Autodesk Inventor part; units mm, degrees
note: some values were not read from the file. Chosen so that the rebuilt part matches the saved one: sketch regions of "Extrusion4".
(part 2 of 2)
sketch "Skizze14" plane through (0, 0, -25) normal (0, 0, -1) x (-1, 0, 0)
  circle A0 centre (0, 0) radius 27.4555 construction
  circle A1 centre (0, 0) radius 26.4655
  circle A2 centre (0, 0) radius 29.1655 construction
  circle A3 centre (0, 0) radius 27.2155 construction
  line L0 (-1.465, 27.176) -> (1.465, 27.176) construction
  line L1 (3.028, 27.0465) -> (5.918, 26.5643) construction
  arc A4 (4.0071, 28.7853) -> (3.1451, 27.5107) centre (5.918, 26.5643) ccw
  arc A5 (0.5608, 29.1601) -> (0, 29.1655) centre (0, 0) ccw
  arc A6 (4.8005, 28.7677) -> (4.2464, 28.8547) centre (0, 0) ccw
  arc A7 (2.8303, 27.3092) -> (1.7033, 27.4026) centre (0, 0) ccw
  arc A8 (1.4259, 27.6532) -> (0.7855, 29.0523) centre (-1.465, 27.176) ccw
  arc A9 (0.7855, 29.0523) -> (0.5608, 29.1601) centre (0.5551, 28.8602) ccw
  arc A10 (1.4259, 27.6532) -> (1.7033, 27.4026) centre (1.7219, 27.702) ccw
  arc A11 (2.8303, 27.3092) -> (3.1451, 27.5107) centre (2.8612, 27.6076) ccw
  arc A12 (4.2464, 28.8547) -> (4.0071, 28.7853) centre (4.2027, 28.5579) ccw
  line L2 (-49.6175, 0) -> (49.6175, 0) construction
  line L3 (0, -54.7) -> (0, 48.2) construction
  line L4 (4.8005, 28.7677) -> (0, 0) construction
  line L5 (0, 0) -> (2.5656, 30.9622) construction
  arc A13 (-0.5608, 29.1601) -> (-0.7855, 29.0523) centre (-0.5551, 28.8602) ccw
  arc A14 (-0.7855, 29.0523) -> (-1.4259, 27.6532) centre (1.465, 27.176) ccw
  arc A15 (-1.7033, 27.4026) -> (-1.4259, 27.6532) centre (-1.7219, 27.702) ccw
  arc A16 (-3.1451, 27.5107) -> (-2.8303, 27.3092) centre (-2.8612, 27.6076) ccw
  arc A17 (-3.1451, 27.5107) -> (-4.0071, 28.7853) centre (-5.918, 26.5643) ccw
  arc A18 (-4.0071, 28.7853) -> (-4.2464, 28.8547) centre (-4.2027, 28.5579) ccw
  arc A19 (0, 29.1655) -> (-0.5608, 29.1601) centre (0, 0) ccw
  arc A20 (-4.2464, 28.8547) -> (-4.8005, 28.7677) centre (0, 0) ccw
  arc A21 (-1.7033, 27.4026) -> (-2.8303, 27.3092) centre (0, 0) ccw
  arc A22 (-5.3528, 28.6701) -> (-5.5566, 28.5267) centre (-5.2977, 28.3752) ccw
  arc A23 (-5.5566, 28.5267) -> (-5.958, 27.0413) centre (-3.028, 27.0465) ccw
  arc A24 (-6.1904, 26.7485) -> (-5.958, 27.0413) centre (-6.258, 27.0408) ccw
  arc A25 (-7.6303, 26.6178) -> (-7.2866, 26.4709) centre (-7.3662, 26.7602) ccw
  arc A26 (-7.6303, 26.6178) -> (-8.6903, 27.7332) centre (-10.2097, 25.2279) ccw
  arc A27 (-8.6903, 27.7332) -> (-8.9378, 27.7622) centre (-8.8459, 27.4767) ccw
  arc A28 (-4.8005, 28.7677) -> (-5.3528, 28.6701) centre (0, 0) ccw
  arc A29 (-8.9378, 27.7622) -> (-9.47, 27.5852) centre (0, 0) ccw
  arc A30 (-6.1904, 26.7485) -> (-7.2866, 26.4709) centre (0, 0) ccw
  arc A31 (-9.9987, 27.398) -> (-10.1762, 27.2231) centre (-9.8959, 27.1162) ccw
  arc A32 (-10.1762, 27.2231) -> (-10.3276, 25.6919) centre (-7.4384, 26.1792) ccw
  arc A33 (-10.5086, 25.3648) -> (-10.3276, 25.6919) centre (-10.6234, 25.642) ccw
  arc A34 (-11.9074, 24.9989) -> (-11.5442, 24.9105) centre (-11.6704, 25.1827) ccw
  arc A35 (-11.9074, 24.9989) -> (-13.1365, 25.9246) centre (-14.2228, 23.2033) ccw
  arc A36 (-13.1365, 25.9246) -> (-13.3854, 25.9125) centre (-13.2478, 25.6459) ccw
  arc A37 (-9.47, 27.5852) -> (-9.9987, 27.398) centre (0, 0) ccw
  arc A38 (-13.3854, 25.9125) -> (-13.8812, 25.6503) centre (0, 0) ccw
  arc A39 (-10.5086, 25.3648) -> (-11.5442, 24.9105) centre (0, 0) ccw
  arc A40 (-14.3719, 25.3786) -> (-14.5182, 25.1769) centre (-14.2241, 25.1176) ccw
  arc A41 (-14.5182, 25.1769) -> (-14.4155, 23.6416) centre (-11.6459, 24.5979) ccw
  arc A42 (-14.5402, 23.2892) -> (-14.4155, 23.6416) centre (-14.6991, 23.5437) ccw
  arc A43 (-15.8597, 22.698) -> (-15.4869, 22.6707) centre (-15.6561, 22.9184) ccw
  arc A44 (-15.8597, 22.698) -> (-17.2244, 23.4088) centre (-17.848, 20.5459) ccw
  arc A45 (-17.2244, 23.4088) -> (-17.4679, 23.3559) centre (-17.2883, 23.1156) ccw
  arc A46 (-13.8812, 25.6503) -> (-14.3719, 25.3786) centre (0, 0) ccw
  arc A47 (-17.4679, 23.3559) -> (-17.9138, 23.0157) centre (0, 0) ccw
  arc A48 (-14.5402, 23.2892) -> (-15.4869, 22.6707) centre (0, 0) ccw
  arc A49 (-18.3531, 22.667) -> (-18.4641, 22.4439) centre (-18.1643, 22.4338) ccw
  arc A50 (-18.4641, 22.4439) -> (-18.1102, 20.9464) centre (-15.5358, 22.3455) ccw
  arc A51 (-18.1752, 20.5783) -> (-18.1102, 20.9464) centre (-18.3737, 20.8032) ccw
  arc A52 (-19.3794, 19.778) -> (-19.0072, 19.8124) centre (-19.2148, 20.0289) ccw
  arc A53 (-19.3794, 19.778) -> (-20.8425, 20.2545) centre (-20.9863, 17.328) ccw
  arc A54 (-20.8425, 20.2545) -> (-21.0739, 20.1622) centre (-20.8572, 19.9548) ccw
  arc A55 (-17.9138, 23.0157) -> (-18.3531, 22.667) centre (0, 0) ccw
  arc A56 (-21.0739, 20.1622) -> (-21.4578, 19.7533) centre (0, 0) ccw
  arc A57 (-18.1752, 20.5783) -> (-19.0072, 19.8124) centre (0, 0) ccw
  arc A58 (-21.8336, 19.337) -> (-21.9064, 19.0987) centre (-21.609, 19.1381) ccw
  arc A59 (-21.9064, 19.0987) -> (-21.3108, 17.6799) centre (-19.0018, 19.4837) ccw
  arc A60 (-21.3144, 17.3061) -> (-21.3108, 17.6799) centre (-21.5472, 17.4952) ccw
  arc A61 (-22.3704, 16.3186) -> (-22.0089, 16.4137) centre (-22.2494, 16.5931) ccw
  arc A62 (-22.3704, 16.3186) -> (-23.892, 16.5477) centre (-23.5521, 13.6374) ccw
  arc A63 (-23.892, 16.5477) -> (-24.1051, 16.4186) centre (-23.8572, 16.2497) ccw
  arc A64 (-21.4578, 19.7533) -> (-21.8336, 19.337) centre (0, 0) ccw
  arc A65 (-24.1051, 16.4186) -> (-24.4164, 15.952) centre (0, 0) ccw
  arc A66 (-21.3144, 17.3061) -> (-22.0089, 16.4137) centre (0, 0) ccw
  arc A67 (-24.7186, 15.4796) -> (-24.7512, 15.2325) centre (-24.4643, 15.3203) ccw
  arc A68 (-24.7512, 15.2325) -> (-23.9302, 13.9311) centre (-21.9496, 16.0903) ccw
  arc A69 (-23.8721, 13.5619) -> (-23.9302, 13.9311) centre (-24.133, 13.7101) ccw
  arc A70 (-24.7513, 12.4139) -> (-24.4104, 12.5673) centre (-24.6771, 12.7046) ccw
  arc A71 (-24.7513, 12.4139) -> (-26.2898, 12.3895) centre (-25.4756, 9.5749) ccw
  arc A72 (-26.2898, 12.3895) -> (-26.4788, 12.2271) centre (-26.2064, 12.1013) ccw
  arc A73 (-24.4164, 15.952) -> (-24.7186, 15.4796) centre (0, 0) ccw
  arc A74 (-26.4788, 12.2271) -> (-26.709, 11.7156) centre (0, 0) ccw
  arc A75 (-23.8721, 13.5619) -> (-24.4104, 12.5673) centre (0, 0) ccw
  arc A76 (-26.9293, 11.1999) -> (-26.9208, 10.9508) centre (-26.6523, 11.0847) ccw
  arc A77 (-26.9208, 10.9508) -> (-25.8968, 9.8024) centre (-24.2986, 12.2581) ccw
  arc A78 (-25.7788, 9.4477) -> (-25.8968, 9.8024) centre (-26.0605, 9.5509) ccw
  arc A79 (-26.457, 8.1707) -> (-26.146, 8.3781) centre (-26.4317, 8.4696) ccw
  arc A80 (-26.457, 8.1707) -> (-27.9704, 7.8934) centre (-26.7041, 5.2512) ccw
  arc A81 (-27.9704, 7.8934) -> (-28.1301, 7.702) centre (-27.8408, 7.6228) ccw
  arc A82 (-26.709, 11.7156) -> (-26.9293, 11.1999) centre (0, 0) ccw
  arc A83 (-28.1301, 7.702) -> (-28.273, 7.1597) centre (0, 0) ccw
  arc A84 (-25.7788, 9.4477) -> (-26.146, 8.3781) centre (0, 0) ccw
  arc A85 (-28.4055, 6.6147) -> (-28.3561, 6.3705) centre (-28.1133, 6.5467) ccw
  arc A86 (-28.3561, 6.3705) -> (-27.157, 5.4062) centre (-25.9848, 8.0915) ccw
  arc A87 (-26.9822, 5.0758) -> (-27.157, 5.4062) centre (-27.2771, 5.1313) ccw
  arc A88 (-27.441, 3.7046) -> (-27.1684, 3.9603) centre (-27.4652, 4.0036) ccw
  arc A89 (-27.441, 3.7046) -> (-28.8882, 3.1819) centre (-27.2042, 0.7842) ccw
  arc A90 (-28.8882, 3.1819) -> (-29.0142, 2.9669) centre (-28.7157, 2.9364) ccw
  arc A91 (-28.273, 7.1597) -> (-28.4055, 6.6147) centre (0, 0) ccw
  arc A92 (-29.0142, 2.9669) -> (-29.0659, 2.4085) centre (0, 0) ccw
  arc A93 (-26.9822, 5.0758) -> (-27.1684, 3.9603) centre (0, 0) ccw
  arc A94 (-29.1068, 1.8491) -> (-29.0179, 1.6163) centre (-28.8074, 1.8301) ccw
  arc A95 (-29.0179, 1.6163) -> (-27.6765, 0.8626) centre (-26.9622, 3.7042) ccw
  arc A96 (-27.4497, 0.5654) -> (-27.6765, 0.8626) centre (-27.7496, 0.5716) ccw
  arc A97 (-27.6765, -0.8626) -> (-27.4497, -0.5654) centre (-27.7496, -0.5716) ccw
  arc A98 (-27.6765, -0.8626) -> (-29.0179, -1.6163) centre (-26.9622, -3.7042) ccw
  arc A99 (-29.0179, -1.6163) -> (-29.1068, -1.8491) centre (-28.8074, -1.8301) ccw
  arc A100 (-29.0659, 2.4085) -> (-29.1068, 1.8491) centre (0, 0) ccw
  arc A101 (-29.1068, -1.8491) -> (-29.0659, -2.4085) centre (0, 0) ccw
  arc A102 (-27.4497, 0.5654) -> (-27.4497, -0.5654) centre (0, 0) ccw
  arc A103 (-29.0142, -2.9669) -> (-28.8882, -3.1819) centre (-28.7157, -2.9364) ccw
  arc A104 (-28.8882, -3.1819) -> (-27.441, -3.7046) centre (-27.2042, -0.7842) ccw
  arc A105 (-27.1684, -3.9603) -> (-27.441, -3.7046) centre (-27.4652, -4.0036) ccw
  arc A106 (-27.157, -5.4062) -> (-26.9822, -5.0758) centre (-27.2771, -5.1313) ccw
  arc A107 (-27.157, -5.4062) -> (-28.3561, -6.3705) centre (-25.9848, -8.0915) ccw
  arc A108 (-28.3561, -6.3705) -> (-28.4055, -6.6147) centre (-28.1133, -6.5467) ccw
  arc A109 (-29.0659, -2.4085) -> (-29.0142, -2.9669) centre (0, 0) ccw
  arc A110 (-28.4055, -6.6147) -> (-28.273, -7.1597) centre (0, 0) ccw
  arc A111 (-27.1684, -3.9603) -> (-26.9822, -5.0758) centre (0, 0) ccw
  arc A112 (-28.1301, -7.702) -> (-27.9704, -7.8934) centre (-27.8408, -7.6228) ccw
  arc A113 (-27.9704, -7.8934) -> (-26.457, -8.1707) centre (-26.7041, -5.2512) ccw
  arc A114 (-26.146, -8.3781) -> (-26.457, -8.1707) centre (-26.4317, -8.4696) ccw
  arc A115 (-25.8968, -9.8024) -> (-25.7788, -9.4477) centre (-26.0605, -9.5509) ccw
  arc A116 (-25.8968, -9.8024) -> (-26.9208, -10.9508) centre (-24.2986, -12.2581) ccw
  arc A117 (-26.9208, -10.9508) -> (-26.9293, -11.1999) centre (-26.6523, -11.0847) ccw
  arc A118 (-28.273, -7.1597) -> (-28.1301, -7.702) centre (0, 0) ccw
  arc A119 (-26.9293, -11.1999) -> (-26.709, -11.7156) centre (0, 0) ccw
  arc A120 (-26.146, -8.3781) -> (-25.7788, -9.4477) centre (0, 0) ccw
  arc A121 (-26.4788, -12.2271) -> (-26.2898, -12.3895) centre (-26.2064, -12.1013) ccw
  arc A122 (-26.2898, -12.3895) -> (-24.7513, -12.4139) centre (-25.4756, -9.5749) ccw
  arc A123 (-24.4104, -12.5673) -> (-24.7513, -12.4139) centre (-24.6771, -12.7046) ccw
  arc A124 (-23.9302, -13.9311) -> (-23.8721, -13.5619) centre (-24.133, -13.7101) ccw
  arc A125 (-23.9302, -13.9311) -> (-24.7512, -15.2325) centre (-21.9496, -16.0903) ccw
  arc A126 (-24.7512, -15.2325) -> (-24.7186, -15.4796) centre (-24.4643, -15.3203) ccw
  arc A127 (-26.709, -11.7156) -> (-26.4788, -12.2271) centre (0, 0) ccw
  arc A128 (-24.7186, -15.4796) -> (-24.4164, -15.952) centre (0, 0) ccw
  arc A129 (-24.4104, -12.5673) -> (-23.8721, -13.5619) centre (0, 0) ccw
  arc A130 (-24.1051, -16.4186) -> (-23.892, -16.5477) centre (-23.8572, -16.2497) ccw
  arc A131 (-23.892, -16.5477) -> (-22.3704, -16.3186) centre (-23.5521, -13.6374) ccw
  arc A132 (-22.0089, -16.4137) -> (-22.3704, -16.3186) centre (-22.2494, -16.5931) ccw
  arc A133 (-21.3108, -17.6799) -> (-21.3144, -17.3061) centre (-21.5472, -17.4952) ccw
  arc A134 (-21.3108, -17.6799) -> (-21.9064, -19.0987) centre (-19.0018, -19.4837) ccw
  arc A135 (-21.9064, -19.0987) -> (-21.8336, -19.337) centre (-21.609, -19.1381) ccw
  arc A136 (-24.4164, -15.952) -> (-24.1051, -16.4186) centre (0, 0) ccw
  arc A137 (-21.8336, -19.337) -> (-21.4578, -19.7533) centre (0, 0) ccw
  arc A138 (-22.0089, -16.4137) -> (-21.3144, -17.3061) centre (0, 0) ccw
  arc A139 (-21.0739, -20.1622) -> (-20.8425, -20.2545) centre (-20.8572, -19.9548) ccw
  arc A140 (-20.8425, -20.2545) -> (-19.3794, -19.778) centre (-20.9863, -17.328) ccw
  arc A141 (-19.0072, -19.8124) -> (-19.3794, -19.778) centre (-19.2148, -20.0289) ccw
  arc A142 (-18.1102, -20.9464) -> (-18.1752, -20.5783) centre (-18.3737, -20.8032) ccw
  arc A143 (-18.1102, -20.9464) -> (-18.4641, -22.4439) centre (-15.5358, -22.3455) ccw
  arc A144 (-18.4641, -22.4439) -> (-18.3531, -22.667) centre (-18.1643, -22.4338) ccw
  arc A145 (-21.4578, -19.7533) -> (-21.0739, -20.1622) centre (0, 0) ccw
  arc A146 (-18.3531, -22.667) -> (-17.9138, -23.0157) centre (0, 0) ccw
  arc A147 (-19.0072, -19.8124) -> (-18.1752, -20.5783) centre (0, 0) ccw
  arc A148 (-17.4679, -23.3559) -> (-17.2244, -23.4088) centre (-17.2883, -23.1156) ccw
  arc A149 (-17.2244, -23.4088) -> (-15.8597, -22.698) centre (-17.848, -20.5459) ccw
  arc A150 (-15.4869, -22.6707) -> (-15.8597, -22.698) centre (-15.6561, -22.9184) ccw
  arc A151 (-14.4155, -23.6416) -> (-14.5402, -23.2892) centre (-14.6991, -23.5437) ccw
  arc A152 (-14.4155, -23.6416) -> (-14.5182, -25.1769) centre (-11.6459, -24.5979) ccw
  arc A153 (-14.5182, -25.1769) -> (-14.3719, -25.3786) centre (-14.2241, -25.1176) ccw
  arc A154 (-17.9138, -23.0157) -> (-17.4679, -23.3559) centre (0, 0) ccw
  arc A155 (-14.3719, -25.3786) -> (-13.8812, -25.6503) centre (0, 0) ccw
  arc A156 (-15.4869, -22.6707) -> (-14.5402, -23.2892) centre (0, 0) ccw
  arc A157 (-13.3854, -25.9125) -> (-13.1365, -25.9246) centre (-13.2478, -25.6459) ccw
  arc A158 (-13.1365, -25.9246) -> (-11.9074, -24.9989) centre (-14.2228, -23.2033) ccw
  arc A159 (-11.5442, -24.9105) -> (-11.9074, -24.9989) centre (-11.6704, -25.1827) ccw
  arc A160 (-10.3276, -25.6919) -> (-10.5086, -25.3648) centre (-10.6234, -25.642) ccw
  arc A161 (-10.3276, -25.6919) -> (-10.1762, -27.2231) centre (-7.4384, -26.1792) ccw
  arc A162 (-10.1762, -27.2231) -> (-9.9987, -27.398) centre (-9.8959, -27.1162) ccw
  arc A163 (-13.8812, -25.6503) -> (-13.3854, -25.9125) centre (0, 0) ccw
  arc A164 (-9.9987, -27.398) -> (-9.47, -27.5852) centre (0, 0) ccw
  arc A165 (-11.5442, -24.9105) -> (-10.5086, -25.3648) centre (0, 0) ccw
  arc A166 (-8.9378, -27.7622) -> (-8.6903, -27.7332) centre (-8.8459, -27.4767) ccw
  arc A167 (-8.6903, -27.7332) -> (-7.6303, -26.6178) centre (-10.2097, -25.2279) ccw
  arc A168 (-7.2866, -26.4709) -> (-7.6303, -26.6178) centre (-7.3662, -26.7602) ccw
  arc A169 (-5.958, -27.0413) -> (-6.1904, -26.7485) centre (-6.258, -27.0408) ccw
  arc A170 (-5.958, -27.0413) -> (-5.5566, -28.5267) centre (-3.028, -27.0465) ccw
  arc A171 (-5.5566, -28.5267) -> (-5.3528, -28.6701) centre (-5.2977, -28.3752) ccw
  arc A172 (-9.47, -27.5852) -> (-8.9378, -27.7622) centre (0, 0) ccw
  arc A173 (-5.3528, -28.6701) -> (-4.8005, -28.7677) centre (0, 0) ccw
  arc A174 (-7.2866, -26.4709) -> (-6.1904, -26.7485) centre (0, 0) ccw
  arc A175 (-4.2464, -28.8547) -> (-4.0071, -28.7853) centre (-4.2027, -28.5579) ccw
  arc A176 (-4.0071, -28.7853) -> (-3.1451, -27.5107) centre (-5.918, -26.5643) ccw
  arc A177 (-2.8303, -27.3092) -> (-3.1451, -27.5107) centre (-2.8612, -27.6076) ccw
  arc A178 (-1.4259, -27.6532) -> (-1.7033, -27.4026) centre (-1.7219, -27.702) ccw
  arc A179 (-1.4259, -27.6532) -> (-0.7855, -29.0523) centre (1.465, -27.176) ccw
  arc A180 (-0.7855, -29.0523) -> (-0.5608, -29.1601) centre (-0.5551, -28.8602) ccw
  arc A181 (-4.8005, -28.7677) -> (-4.2464, -28.8547) centre (0, 0) ccw
  arc A182 (-0.5608, -29.1601) -> (0, -29.1655) centre (0, 0) ccw
  arc A183 (-2.8303, -27.3092) -> (-1.7033, -27.4026) centre (0, 0) ccw
  arc A184 (0.5608, -29.1601) -> (0.7855, -29.0523) centre (0.5551, -28.8602) ccw
  arc A185 (0.7855, -29.0523) -> (1.4259, -27.6532) centre (-1.465, -27.176) ccw
  arc A186 (1.7033, -27.4026) -> (1.4259, -27.6532) centre (1.7219, -27.702) ccw
  arc A187 (3.1451, -27.5107) -> (2.8303, -27.3092) centre (2.8612, -27.6076) ccw
  arc A188 (3.1451, -27.5107) -> (4.0071, -28.7853) centre (5.918, -26.5643) ccw
  arc A189 (4.0071, -28.7853) -> (4.2464, -28.8547) centre (4.2027, -28.5579) ccw
  arc A190 (0, -29.1655) -> (0.5608, -29.1601) centre (0, 0) ccw
  arc A191 (4.2464, -28.8547) -> (4.8005, -28.7677) centre (0, 0) ccw
  arc A192 (1.7033, -27.4026) -> (2.8303, -27.3092) centre (0, 0) ccw
  arc A193 (5.3528, -28.6701) -> (5.5566, -28.5267) centre (5.2977, -28.3752) ccw
  arc A194 (5.5566, -28.5267) -> (5.958, -27.0413) centre (3.028, -27.0465) ccw
  arc A195 (6.1904, -26.7485) -> (5.958, -27.0413) centre (6.258, -27.0408) ccw
  arc A196 (7.6303, -26.6178) -> (7.2866, -26.4709) centre (7.3662, -26.7602) ccw
  arc A197 (7.6303, -26.6178) -> (8.6903, -27.7332) centre (10.2097, -25.2279) ccw
  arc A198 (8.6903, -27.7332) -> (8.9378, -27.7622) centre (8.8459, -27.4767) ccw
  arc A199 (4.8005, -28.7677) -> (5.3528, -28.6701) centre (0, 0) ccw
  arc A200 (8.9378, -27.7622) -> (9.47, -27.5852) centre (0, 0) ccw
  arc A201 (6.1904, -26.7485) -> (7.2866, -26.4709) centre (0, 0) ccw
  arc A202 (9.9987, -27.398) -> (10.1762, -27.2231) centre (9.8959, -27.1162) ccw
  arc A203 (10.1762, -27.2231) -> (10.3276, -25.6919) centre (7.4384, -26.1792) ccw
  arc A204 (10.5086, -25.3648) -> (10.3276, -25.6919) centre (10.6234, -25.642) ccw
  arc A205 (11.9074, -24.9989) -> (11.5442, -24.9105) centre (11.6704, -25.1827) ccw
  arc A206 (11.9074, -24.9989) -> (13.1365, -25.9246) centre (14.2228, -23.2033) ccw
  arc A207 (13.1365, -25.9246) -> (13.3854, -25.9125) centre (13.2478, -25.6459) ccw
  arc A208 (9.47, -27.5852) -> (9.9987, -27.398) centre (0, 0) ccw
  arc A209 (13.3854, -25.9125) -> (13.8812, -25.6503) centre (0, 0) ccw
  arc A210 (10.5086, -25.3648) -> (11.5442, -24.9105) centre (0, 0) ccw
  arc A211 (14.3719, -25.3786) -> (14.5182, -25.1769) centre (14.2241, -25.1176) ccw
  arc A212 (14.5182, -25.1769) -> (14.4155, -23.6416) centre (11.6459, -24.5979) ccw
  arc A213 (14.5402, -23.2892) -> (14.4155, -23.6416) centre (14.6991, -23.5437) ccw
  arc A214 (15.8597, -22.698) -> (15.4869, -22.6707) centre (15.6561, -22.9184) ccw
  arc A215 (15.8597, -22.698) -> (17.2244, -23.4088) centre (17.848, -20.5459) ccw
  arc A216 (17.2244, -23.4088) -> (17.4679, -23.3559) centre (17.2883, -23.1156) ccw
  arc A217 (13.8812, -25.6503) -> (14.3719, -25.3786) centre (0, 0) ccw
  arc A218 (17.4679, -23.3559) -> (17.9138, -23.0157) centre (0, 0) ccw
  arc A219 (14.5402, -23.2892) -> (15.4869, -22.6707) centre (0, 0) ccw
  arc A220 (18.3531, -22.667) -> (18.4641, -22.4439) centre (18.1643, -22.4338) ccw
  arc A221 (18.4641, -22.4439) -> (18.1102, -20.9464) centre (15.5358, -22.3455) ccw
  arc A222 (18.1752, -20.5783) -> (18.1102, -20.9464) centre (18.3737, -20.8032) ccw
  arc A223 (19.3794, -19.778) -> (19.0072, -19.8124) centre (19.2148, -20.0289) ccw
  arc A224 (19.3794, -19.778) -> (20.8425, -20.2545) centre (20.9863, -17.328) ccw
  arc A225 (20.8425, -20.2545) -> (21.0739, -20.1622) centre (20.8572, -19.9548) ccw
  arc A226 (17.9138, -23.0157) -> (18.3531, -22.667) centre (0, 0) ccw
  arc A227 (21.0739, -20.1622) -> (21.4578, -19.7533) centre (0, 0) ccw
  arc A228 (18.1752, -20.5783) -> (19.0072, -19.8124) centre (0, 0) ccw
  arc A229 (21.8336, -19.337) -> (21.9064, -19.0987) centre (21.609, -19.1381) ccw
  arc A230 (21.9064, -19.0987) -> (21.3108, -17.6799) centre (19.0018, -19.4837) ccw
  arc A231 (21.3144, -17.3061) -> (21.3108, -17.6799) centre (21.5472, -17.4952) ccw
  arc A232 (22.3704, -16.3186) -> (22.0089, -16.4137) centre (22.2494, -16.5931) ccw
  arc A233 (22.3704, -16.3186) -> (23.892, -16.5477) centre (23.5521, -13.6374) ccw
  arc A234 (23.892, -16.5477) -> (24.1051, -16.4186) centre (23.8572, -16.2497) ccw
  arc A235 (21.4578, -19.7533) -> (21.8336, -19.337) centre (0, 0) ccw
  arc A236 (24.1051, -16.4186) -> (24.4164, -15.952) centre (0, 0) ccw
  arc A237 (21.3144, -17.3061) -> (22.0089, -16.4137) centre (0, 0) ccw
  arc A238 (24.7186, -15.4796) -> (24.7512, -15.2325) centre (24.4643, -15.3203) ccw
  arc A239 (24.7512, -15.2325) -> (23.9302, -13.9311) centre (21.9496, -16.0903) ccw
  arc A240 (23.8721, -13.5619) -> (23.9302, -13.9311) centre (24.133, -13.7101) ccw
  arc A241 (24.7513, -12.4139) -> (24.4104, -12.5673) centre (24.6771, -12.7046) ccw
  arc A242 (24.7513, -12.4139) -> (26.2898, -12.3895) centre (25.4756, -9.5749) ccw
  arc A243 (26.2898, -12.3895) -> (26.4788, -12.2271) centre (26.2064, -12.1013) ccw
  arc A244 (24.4164, -15.952) -> (24.7186, -15.4796) centre (0, 0) ccw
  arc A245 (26.4788, -12.2271) -> (26.709, -11.7156) centre (0, 0) ccw
  arc A246 (23.8721, -13.5619) -> (24.4104, -12.5673) centre (0, 0) ccw
  arc A247 (26.9293, -11.1999) -> (26.9208, -10.9508) centre (26.6523, -11.0847) ccw
  arc A248 (26.9208, -10.9508) -> (25.8968, -9.8024) centre (24.2986, -12.2581) ccw
  arc A249 (25.7788, -9.4477) -> (25.8968, -9.8024) centre (26.0605, -9.5509) ccw
  arc A250 (26.457, -8.1707) -> (26.146, -8.3781) centre (26.4317, -8.4696) ccw
  arc A251 (26.457, -8.1707) -> (27.9704, -7.8934) centre (26.7041, -5.2512) ccw
  arc A252 (27.9704, -7.8934) -> (28.1301, -7.702) centre (27.8408, -7.6228) ccw
  arc A253 (26.709, -11.7156) -> (26.9293, -11.1999) centre (0, 0) ccw
  arc A254 (28.1301, -7.702) -> (28.273, -7.1597) centre (0, 0) ccw
  arc A255 (25.7788, -9.4477) -> (26.146, -8.3781) centre (0, 0) ccw
  arc A256 (28.4055, -6.6147) -> (28.3561, -6.3705) centre (28.1133, -6.5467) ccw
  arc A257 (28.3561, -6.3705) -> (27.157, -5.4062) centre (25.9848, -8.0915) ccw
  arc A258 (26.9822, -5.0758) -> (27.157, -5.4062) centre (27.2771, -5.1313) ccw
  arc A259 (27.441, -3.7046) -> (27.1684, -3.9603) centre (27.4652, -4.0036) ccw
  arc A260 (27.441, -3.7046) -> (28.8882, -3.1819) centre (27.2042, -0.7842) ccw
  arc A261 (28.8882, -3.1819) -> (29.0142, -2.9669) centre (28.7157, -2.9364) ccw
  arc A262 (28.273, -7.1597) -> (28.4055, -6.6147) centre (0, 0) ccw
  arc A263 (29.0142, -2.9669) -> (29.0659, -2.4085) centre (0, 0) ccw
  arc A264 (26.9822, -5.0758) -> (27.1684, -3.9603) centre (0, 0) ccw
  arc A265 (29.1068, -1.8491) -> (29.0179, -1.6163) centre (28.8074, -1.8301) ccw
  arc A266 (29.0179, -1.6163) -> (27.6765, -0.8626) centre (26.9622, -3.7042) ccw
  arc A267 (27.4497, -0.5654) -> (27.6765, -0.8626) centre (27.7496, -0.5716) ccw
  arc A268 (27.6765, 0.8626) -> (27.4497, 0.5654) centre (27.7496, 0.5716) ccw
  arc A269 (27.6765, 0.8626) -> (29.0179, 1.6163) centre (26.9622, 3.7042) ccw
  arc A270 (29.0179, 1.6163) -> (29.1068, 1.8491) centre (28.8074, 1.8301) ccw
  arc A271 (29.0659, -2.4085) -> (29.1068, -1.8491) centre (0, 0) ccw
  arc A272 (29.1068, 1.8491) -> (29.0659, 2.4085) centre (0, 0) ccw
  arc A273 (27.4497, -0.5654) -> (27.4497, 0.5654) centre (0, 0) ccw
  arc A274 (29.0142, 2.9669) -> (28.8882, 3.1819) centre (28.7157, 2.9364) ccw
  arc A275 (28.8882, 3.1819) -> (27.441, 3.7046) centre (27.2042, 0.7842) ccw
  arc A276 (27.1684, 3.9603) -> (27.441, 3.7046) centre (27.4652, 4.0036) ccw
  arc A277 (27.157, 5.4062) -> (26.9822, 5.0758) centre (27.2771, 5.1313) ccw
  arc A278 (27.157, 5.4062) -> (28.3561, 6.3705) centre (25.9848, 8.0915) ccw
  arc A279 (28.3561, 6.3705) -> (28.4055, 6.6147) centre (28.1133, 6.5467) ccw
  arc A280 (29.0659, 2.4085) -> (29.0142, 2.9669) centre (0, 0) ccw
  arc A281 (28.4055, 6.6147) -> (28.273, 7.1597) centre (0, 0) ccw
  arc A282 (27.1684, 3.9603) -> (26.9822, 5.0758) centre (0, 0) ccw
  arc A283 (28.1301, 7.702) -> (27.9704, 7.8934) centre (27.8408, 7.6228) ccw
  arc A284 (27.9704, 7.8934) -> (26.457, 8.1707) centre (26.7041, 5.2512) ccw
  arc A285 (26.146, 8.3781) -> (26.457, 8.1707) centre (26.4317, 8.4696) ccw
  arc A286 (25.8968, 9.8024) -> (25.7788, 9.4477) centre (26.0605, 9.5509) ccw
  arc A287 (25.8968, 9.8024) -> (26.9208, 10.9508) centre (24.2986, 12.2581) ccw
  arc A288 (26.9208, 10.9508) -> (26.9293, 11.1999) centre (26.6523, 11.0847) ccw
  arc A289 (28.273, 7.1597) -> (28.1301, 7.702) centre (0, 0) ccw
  arc A290 (26.9293, 11.1999) -> (26.709, 11.7156) centre (0, 0) ccw
  arc A291 (26.146, 8.3781) -> (25.7788, 9.4477) centre (0, 0) ccw
  arc A292 (26.4788, 12.2271) -> (26.2898, 12.3895) centre (26.2064, 12.1013) ccw
  arc A293 (26.2898, 12.3895) -> (24.7513, 12.4139) centre (25.4756, 9.5749) ccw
  arc A294 (24.4104, 12.5673) -> (24.7513, 12.4139) centre (24.6771, 12.7046) ccw
  arc A295 (23.9302, 13.9311) -> (23.8721, 13.5619) centre (24.133, 13.7101) ccw
  arc A296 (23.9302, 13.9311) -> (24.7512, 15.2325) centre (21.9496, 16.0903) ccw
  arc A297 (24.7512, 15.2325) -> (24.7186, 15.4796) centre (24.4643, 15.3203) ccw
  arc A298 (26.709, 11.7156) -> (26.4788, 12.2271) centre (0, 0) ccw
  arc A299 (24.7186, 15.4796) -> (24.4164, 15.952) centre (0, 0) ccw
  arc A300 (24.4104, 12.5673) -> (23.8721, 13.5619) centre (0, 0) ccw
  arc A301 (24.1051, 16.4186) -> (23.892, 16.5477) centre (23.8572, 16.2497) ccw
  arc A302 (23.892, 16.5477) -> (22.3704, 16.3186) centre (23.5521, 13.6374) ccw
  arc A303 (22.0089, 16.4137) -> (22.3704, 16.3186) centre (22.2494, 16.5931) ccw
  arc A304 (21.3108, 17.6799) -> (21.3144, 17.3061) centre (21.5472, 17.4952) ccw
  arc A305 (21.3108, 17.6799) -> (21.9064, 19.0987) centre (19.0018, 19.4837) ccw
  arc A306 (21.9064, 19.0987) -> (21.8336, 19.337) centre (21.609, 19.1381) ccw
  arc A307 (24.4164, 15.952) -> (24.1051, 16.4186) centre (0, 0) ccw
  arc A308 (21.8336, 19.337) -> (21.4578, 19.7533) centre (0, 0) ccw
  arc A309 (22.0089, 16.4137) -> (21.3144, 17.3061) centre (0, 0) ccw
  arc A310 (21.0739, 20.1622) -> (20.8425, 20.2545) centre (20.8572, 19.9548) ccw
  arc A311 (20.8425, 20.2545) -> (19.3794, 19.778) centre (20.9863, 17.328) ccw
  arc A312 (19.0072, 19.8124) -> (19.3794, 19.778) centre (19.2148, 20.0289) ccw
  arc A313 (18.1102, 20.9464) -> (18.1752, 20.5783) centre (18.3737, 20.8032) ccw
  arc A314 (18.1102, 20.9464) -> (18.4641, 22.4439) centre (15.5358, 22.3455) ccw
  arc A315 (18.4641, 22.4439) -> (18.3531, 22.667) centre (18.1643, 22.4338) ccw
  arc A316 (21.4578, 19.7533) -> (21.0739, 20.1622) centre (0, 0) ccw
  arc A317 (18.3531, 22.667) -> (17.9138, 23.0157) centre (0, 0) ccw
  arc A318 (19.0072, 19.8124) -> (18.1752, 20.5783) centre (0, 0) ccw
  arc A319 (17.4679, 23.3559) -> (17.2244, 23.4088) centre (17.2883, 23.1156) ccw
  arc A320 (17.2244, 23.4088) -> (15.8597, 22.698) centre (17.848, 20.5459) ccw
  arc A321 (15.4869, 22.6707) -> (15.8597, 22.698) centre (15.6561, 22.9184) ccw
  arc A322 (14.4155, 23.6416) -> (14.5402, 23.2892) centre (14.6991, 23.5437) ccw
  arc A323 (14.4155, 23.6416) -> (14.5182, 25.1769) centre (11.6459, 24.5979) ccw
  arc A324 (14.5182, 25.1769) -> (14.3719, 25.3786) centre (14.2241, 25.1176) ccw
  arc A325 (17.9138, 23.0157) -> (17.4679, 23.3559) centre (0, 0) ccw
  arc A326 (14.3719, 25.3786) -> (13.8812, 25.6503) centre (0, 0) ccw
  arc A327 (15.4869, 22.6707) -> (14.5402, 23.2892) centre (0, 0) ccw
  arc A328 (13.3854, 25.9125) -> (13.1365, 25.9246) centre (13.2478, 25.6459) ccw
  arc A329 (13.1365, 25.9246) -> (11.9074, 24.9989) centre (14.2228, 23.2033) ccw
  arc A330 (11.5442, 24.9105) -> (11.9074, 24.9989) centre (11.6704, 25.1827) ccw
  arc A331 (10.3276, 25.6919) -> (10.5086, 25.3648) centre (10.6234, 25.642) ccw
  arc A332 (10.3276, 25.6919) -> (10.1762, 27.2231) centre (7.4384, 26.1792) ccw
  arc A333 (10.1762, 27.2231) -> (9.9987, 27.398) centre (9.8959, 27.1162) ccw
  arc A334 (13.8812, 25.6503) -> (13.3854, 25.9125) centre (0, 0) ccw
  arc A335 (9.9987, 27.398) -> (9.47, 27.5852) centre (0, 0) ccw
  arc A336 (11.5442, 24.9105) -> (10.5086, 25.3648) centre (0, 0) ccw
  arc A337 (8.9378, 27.7622) -> (8.6903, 27.7332) centre (8.8459, 27.4767) ccw
  arc A338 (8.6903, 27.7332) -> (7.6303, 26.6178) centre (10.2097, 25.2279) ccw
  arc A339 (7.2866, 26.4709) -> (7.6303, 26.6178) centre (7.3662, 26.7602) ccw
  arc A340 (5.958, 27.0413) -> (6.1904, 26.7485) centre (6.258, 27.0408) ccw
  arc A341 (5.958, 27.0413) -> (5.5566, 28.5267) centre (3.028, 27.0465) ccw
  arc A342 (5.5566, 28.5267) -> (5.3528, 28.6701) centre (5.2977, 28.3752) ccw
  arc A343 (9.47, 27.5852) -> (8.9378, 27.7622) centre (0, 0) ccw
  arc A344 (5.3528, 28.6701) -> (4.8005, 28.7677) centre (0, 0) ccw
  arc A345 (7.2866, 26.4709) -> (6.1904, 26.7485) centre (0, 0) ccw
  circle A346 centre (0, 0) radius 30.6655
  circle A347 centre (0, 0) radius 2
  circle A348 centre (0, 0) radius 6.35 construction
  circle A349 centre (0, 6.35) radius 1.5
  circle A350 centre (-6.35, 0) radius 1.5
  circle A351 centre (0, -6.35) radius 1.5
  circle A352 centre (6.35, 0) radius 1.5
  dimension "d298" = 12.7
  dimension "d273" = 1.71
  dimension "d274" = 2.7
  dimension "d275" = 0.75
  dimension "d276" = 54.431
  dimension "d277" = 2.93
  dimension "d278" = 0.3
  dimension "d279" = 2.93
  dimension "d280" = 9.474
  dimension "d291" = 1.5
  dimension "d292" = 4
  dimension "d293" = 3
  dimension "d296" = 360
  constraints: 694 point on circle, 352 centre point, 8 coincident, 8 end point, 8 tangent, 6 equal radius, 2 point on line, 1 equal length, 1 horizontal, 1 vertical alignment, 13 other
  measures "d273" radial gap between concentric circles of A2 A0
  measures "d274" radial gap between concentric circles of A2 A1
  measures "d275" radial gap between concentric circles of A3 A1
  measures "d276" diameter of A3
  measures "d277" distance of L0.start L0.end
  measures "d278" radius of A9
  measures "d279" radius of A8
  measures "d280" angle of L3 L4
  measures "d291" radial gap between concentric circles of A346 A2
  measures "d292" diameter of A347
  measures "d293" diameter of A349
extrude "Extrusion34" add sketch "Skizze14" against normal blind 2 separate body contours A1 | A12 A6 A344 A342 A341 A340 A345 A339 A338 A337 A343 A335 A333 A332 A331 A336 A330 A329 A328 A334 A326 A324 A323 A322 A327 A321 A320 A319 A325 A317 A315 A314 A313 A318 A312 A311 A310 A316 A308 A306 A305 A304 A309 A303 A302 A301 A307 A299 A297 A296 A295 A300 A294 A293 A292 A298 A290 A288 A287 A286 A291 A285 A284 A283 A289 A281 A279 A278 A277 A282 A276 A275 A274 A280 A272 A270 A269 A268 A273 A267 A266 A265 A271 A263 A261 A260 A259 A264 A258 A257 A256 A262 A254 A252 A251 A250 A255 A249 A248 A247 A253 A245 A243 A242 A241 A246 A240 A239 A238 A244 A236 A234 A233 A232 A237 A231 A230 A229 A235 A227 A225 A224 A223 A228 A222 A221 A220 A226 A218 A216 A215 A214 A219 A213 A212 A211 A217 A209 A207 A206 A205 A210 A204 A203 A202 A208 A200 A198 A197 A196 A201 A195 A194 A193 A199 A191 A189 A188 A187 A192 A186 A185 A184 A190 A182 A180 A179 A178 A183 A177 A176 A175 A181 A173 A171 A170 A169 A174 A168 A167 A166 A172 A164 A162 A161 A160 A165 A159 A158 A157 A163 A155 A153 A152 A151 A156 A150 A149 A148 A154 A146 A144 A143 A142 A147 A141 A140 A139 A145 A137 A135 A134 A133 A138 A132 A131 A130 A136 A128 A126 A125 A124 A129 A123 A122 A121 A127 A119 A117 A116 A115 A120 A114 A113 A112 A118 A110 A108 A107 A106 A111 A105 A104 A103 A109 A101 A99 A98 A97 A102 A96 A95 A94 A100 A92 A90 A89 A88 A93 A87 A86 A85 A91 A83 A81 A80 A79 A84 A78 A77 A76 A82 A74 A72 A71 A70 A75 A69 A68 A67 A73 A65 A63 A62 A61 A66 A60 A59 A58 A64 A56 A54 A53 A52 A57 A51 A50 A49 A55 A47 A45 A44 A43 A48 A42 A41 A40 A46 A38 A36 A35 A34 A39 A33 A32 A31 A37 A29 A27 A26 A25 A30 A24 A23 A22 A28 A20 A18 A17 A16 A21 A15 A14 A13 A19 A5 A9 A8 A10 A7 A11 A4 | A346
extrude "Extrusion35" add sketch "Skizze14" against normal blind 7 contours A346 bodies 3
